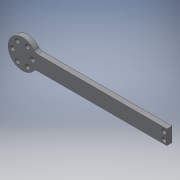
# Autodesk Inventor part: test_arm_2
Saved by Autodesk Inventor 2019.4 (Build 234330000, 330)
## iProperties
Created: 2019-08-15
Part Number: test_arm_2
Material: 일반
Document SubType Name: Modeling
Designer: cdi
Density: 1 g/cm^3
Appearance: 기본값
Author: cdi
Autodesk Inventor part; units mm, degrees
ref_plane "YZ Plane" through (0, 0, 0) normal (1, 0, 0) x (0, 1, 0)
ref_plane "XZ Plane" through (0, 0, 0) normal (0, 1, 0) x (-1, 0, 0)
ref_plane "XY Plane" through (0, 0, 0) normal (0, 0, 1) x (1, 0, 0)
sketch "스케치1" plane through (0, 0, 0) normal (0, 0, 1) x (1, 0, 0)
  circle A0 centre (0, 0) radius 20
  dimension "d0" = 40
  constraints: 1 centre point, 1 coincident
  measures "d0" diameter of A0
extrude "돌출1" add sketch "스케치1" along normal blind 7
sketch "스케치2" plane through (0, 0, 7) normal (0, 0, 1) x (1, 0, 0)
  circle A0 centre (0, 0) radius 20 projected
  line L0 (17.3205, 10) -> (17.3205, -10)
  line L1 (17.3205, -10) -> (200, -10)
  line L2 (200, -10) -> (200, 10)
  line L3 (200, 10) -> (17.3205, 10)
  dimension "d4" = 10
  dimension "d5" = 20
  dimension "d8" = 200
  constraints: 8 end point, 2 parallel, 2 point on circle, 1 perpendicular, 1 vertical
  measures "d4" distance from line of point (0, 0) L1
  measures "d5" distance of L0.start L0.end
  measures "d8" distance from line of point (0, 0) L2
extrude "돌출2" add sketch "스케치2" against normal blind 7 contours A0 L3 L2 L1
sketch "스케치3" plane through (0, 0, 7) normal (0, 0, 1) x (1, 0, 0)
  circle A0 centre (0, 0) radius 14
  circle A1 centre (14, 0) radius 1.55
  dimension "d9" = 28
  dimension "d10" = 3.1
  constraints: 1 centre point, 1 coincident, 1 horizontal alignment, 2 other
  measures "d10" diameter of A1
hole "구멍1" at (14, 0, 7) direction (0, 0, -1) diameter 3.1 depth 20 countersink diameter 6.5 countersink angle 90
pattern_circular "원형 패턴1" count 6 over 360 about axis through (0, 0, 0) along (0, 0, 1) of "구멍1"
fillet "모깎기1" radius 6 2 edges at (17.3205, 10, 3.5) (17.3205, -10, 3.5)
sketch "스케치4" plane through (0, 0, 7) normal (0, 0, 1) x (1, 0, 0)
  line L0 (20.4939, -10) -> (200, -10) projected
  line L1 (20.4939, 10) -> (200, 10) projected
  line L2 (200, -10) -> (192, -10)
  line L3 (192, -10) -> (192, 10)
  line L4 (192, 10) -> (200, 10)
  line L5 (200, 10) -> (200, -10)
  line L6 (196, 10) -> (196, -10)
  circle A0 centre (196, 5) radius 1.5
  circle A1 centre (196, -5) radius 1.5
  point P0 (0, 0)
  dimension "d22" = 8
  dimension "d23" = 3
  dimension "d24" = 3
  dimension "d25" = 5
  dimension "d26" = 10
  dimension "d27" = 5
  constraints: 10 end point, 3 point on line, 2 centre point, 2 midpoint, 2 parallel, 1 horizontal, 1 perpendicular
  measures "d22" distance of L3.end L4.end
  measures "d23" diameter of A0
  measures "d24" diameter of A1
  measures "d25" distance from line of L0 A1.centre
  measures "d26" distance of A1.centre A0.centre
  measures "d27" distance from line of L1 A0.centre
hole "구멍2" at (196, 5, 7) at (196, -5, 7) direction (0, 0, -1) diameter 3.1 depth 20 countersink diameter 6.5 countersink angle 90
